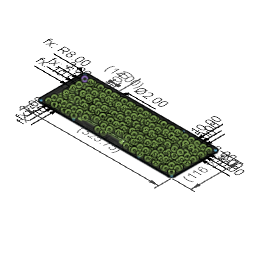
KeychronK6_Case (Autodesk Fusion 360 design; units mm, degrees)
Autodesk Fusion 360 part; units mm, degrees
(part 1 of 4)
sketch "switch-plate" plane through (0, 0, 0) normal (0, 0, 1) x (1, 0, 0) in component "switch-plate"
  spline S0 degree 3 poles (280.7, -89.8) (280.7, -89.9104) (280.6104, -90) (280.5, -90) knots 0 0 0 0 1 1 1 1
  line L0 (280.5, -90) -> (266.9, -90)
  spline S1 degree 3 poles (266.9, -90) (266.7896, -90) (266.7, -89.9104) (266.7, -89.8) knots 2 2 2 2 3 3 3 3
  line L1 (266.7, -89.8) -> (266.7, -76.2)
  spline S2 degree 3 poles (266.7, -76.2) (266.7, -76.0895) (266.7896, -76) (266.9, -76) knots 4 4 4 4 5 5 5 5
  line L2 (266.9, -76) -> (280.5, -76)
  spline S3 degree 3 poles (280.5, -76) (280.6104, -76) (280.7, -76.0895) (280.7, -76.2) knots 6 6 6 6 7 7 7 7
  line L3 (280.7, -76.2) -> (280.7, -89.8)
  spline S4 degree 3 poles (299.75, -13.6) (299.75, -13.7104) (299.6604, -13.8) (299.55, -13.8) knots 0 0 0 0 1 1 1 1
  line L4 (299.55, -13.8) -> (285.95, -13.8)
  spline S5 degree 3 poles (285.95, -13.8) (285.8396, -13.8) (285.75, -13.7104) (285.75, -13.6) knots 2 2 2 2 3 3 3 3
  line L5 (285.75, -13.6) -> (285.75, 0)
  spline S6 degree 3 poles (285.75, 0) (285.75, 0.1105) (285.8396, 0.2) (285.95, 0.2) knots 4 4 4 4 5 5 5 5
  line L6 (285.95, 0.2) -> (299.55, 0.2)
  spline S7 degree 3 poles (299.55, 0.2) (299.6604, 0.2) (299.75, 0.1105) (299.75, 0) knots 6 6 6 6 7 7 7 7
  line L7 (299.75, 0) -> (299.75, -13.6)
  spline S8 degree 3 poles (228.3101, -70.75) (228.3101, -70.8604) (228.2205, -70.95) (228.1101, -70.95) knots 0 0 0 0 1 1 1 1
  line L8 (228.1101, -70.95) -> (214.5101, -70.95)
  spline S9 degree 3 poles (214.5101, -70.95) (214.3997, -70.95) (214.3101, -70.8604) (214.3101, -70.75) knots 2 2 2 2 3 3 3 3
  line L9 (214.3101, -70.75) -> (214.3101, -57.15)
  spline S10 degree 3 poles (214.3101, -57.15) (214.3101, -57.0395) (214.3997, -56.95) (214.5101, -56.95) knots 4 4 4 4 5 5 5 5
  line L10 (214.5101, -56.95) -> (228.1101, -56.95)
  spline S11 degree 3 poles (228.1101, -56.95) (228.2205, -56.95) (228.3101, -57.0395) (228.3101, -57.15) knots 6 6 6 6 7 7 7 7
  line L11 (228.3101, -57.15) -> (228.3101, -70.75)
  spline S12 degree 3 poles (261.65, -89.8) (261.65, -89.9104) (261.5604, -90) (261.45, -90) knots 0 0 0 0 1 1 1 1
  line L12 (261.45, -90) -> (247.85, -90)
  spline S13 degree 3 poles (247.85, -90) (247.7396, -90) (247.65, -89.9104) (247.65, -89.8) knots 2 2 2 2 3 3 3 3
  line L13 (247.65, -89.8) -> (247.65, -76.2)
  spline S14 degree 3 poles (247.65, -76.2) (247.65, -76.0895) (247.7396, -76) (247.85, -76) knots 4 4 4 4 5 5 5 5
  line L14 (247.85, -76) -> (261.45, -76)
  spline S15 degree 3 poles (261.45, -76) (261.5604, -76) (261.65, -76.0895) (261.65, -76.2) knots 6 6 6 6 7 7 7 7
  line L15 (261.65, -76.2) -> (261.65, -89.8)
  spline S16 degree 3 poles (242.6, -89.8) (242.6, -89.9104) (242.5104, -90) (242.4, -90) knots 0 0 0 0 1 1 1 1
  line L16 (242.4, -90) -> (228.8, -90)
  spline S17 degree 3 poles (228.8, -90) (228.6896, -90) (228.6, -89.9104) (228.6, -89.8) knots 2 2 2 2 3 3 3 3
  line L17 (228.6, -89.8) -> (228.6, -76.2)
  spline S18 degree 3 poles (228.6, -76.2) (228.6, -76.0895) (228.6896, -76) (228.8, -76) knots 4 4 4 4 5 5 5 5
  line L18 (228.8, -76) -> (242.4, -76)
  spline S19 degree 3 poles (242.4, -76) (242.5104, -76) (242.6, -76.0895) (242.6, -76.2) knots 6 6 6 6 7 7 7 7
  line L19 (242.6, -76.2) -> (242.6, -89.8)
  spline S20 degree 3 poles (280.7, -70.75) (280.7, -70.8604) (280.6104, -70.95) (280.5, -70.95) knots 0 0 0 0 1 1 1 1
  line L20 (280.5, -70.95) -> (266.9, -70.95)
  spline S21 degree 3 poles (266.9, -70.95) (266.7896, -70.95) (266.7, -70.8604) (266.7, -70.75) knots 2 2 2 2 3 3 3 3
  line L21 (266.7, -70.75) -> (266.7, -57.15)
  spline S22 degree 3 poles (266.7, -57.15) (266.7, -57.0395) (266.7896, -56.95) (266.9, -56.95) knots 4 4 4 4 5 5 5 5
  line L22 (266.9, -56.95) -> (280.5, -56.95)
  spline S23 degree 3 poles (280.5, -56.95) (280.6104, -56.95) (280.7, -57.0395) (280.7, -57.15) knots 6 6 6 6 7 7 7 7
  line L23 (280.7, -57.15) -> (280.7, -70.75)
  line L24 (304.75, 13.2) -> (-5, 13.2)
  line L25 (-13, 5.2) -> (-13, -95)
  line L26 (-5, -103) -> (304.75, -103)
  line L27 (312.75, -95) -> (312.75, 5.2)
  spline S24 degree 3 poles (299.75, -32.65) (299.75, -32.7604) (299.6604, -32.85) (299.55, -32.85) knots 0 0 0 0 1 1 1 1
  line L28 (299.55, -32.85) -> (285.95, -32.85)
  spline S25 degree 3 poles (285.95, -32.85) (285.8396, -32.85) (285.75, -32.7604) (285.75, -32.65) knots 2 2 2 2 3 3 3 3
  line L29 (285.75, -32.65) -> (285.75, -19.05)
  spline S26 degree 3 poles (285.75, -19.05) (285.75, -18.9395) (285.8396, -18.85) (285.95, -18.85) knots 4 4 4 4 5 5 5 5
  line L30 (285.95, -18.85) -> (299.55, -18.85)
  spline S27 degree 3 poles (299.55, -18.85) (299.6604, -18.85) (299.75, -18.9395) (299.75, -19.05) knots 6 6 6 6 7 7 7 7
  line L31 (299.75, -19.05) -> (299.75, -32.65)
  spline S28 degree 3 poles (299.75, -70.75) (299.75, -70.8604) (299.6604, -70.95) (299.55, -70.95) knots 0 0 0 0 1 1 1 1
  line L32 (299.55, -70.95) -> (285.95, -70.95)
  spline S29 degree 3 poles (285.95, -70.95) (285.8396, -70.95) (285.75, -70.8604) (285.75, -70.75) knots 2 2 2 2 3 3 3 3
  line L33 (285.75, -70.75) -> (285.75, -57.15)
  spline S30 degree 3 poles (285.75, -57.15) (285.75, -57.0395) (285.8396, -56.95) (285.95, -56.95) knots 4 4 4 4 5 5 5 5
  line L34 (285.95, -56.95) -> (299.55, -56.95)
  spline S31 degree 3 poles (299.55, -56.95) (299.6604, -56.95) (299.75, -57.0395) (299.75, -57.15) knots 6 6 6 6 7 7 7 7
  line L35 (299.75, -57.15) -> (299.75, -70.75)
  spline S32 degree 3 poles (299.75, -89.8) (299.75, -89.9104) (299.6604, -90) (299.55, -90) knots 0 0 0 0 1 1 1 1
  line L36 (299.55, -90) -> (285.95, -90)
  spline S33 degree 3 poles (285.95, -90) (285.8396, -90) (285.75, -89.9104) (285.75, -89.8) knots 2 2 2 2 3 3 3 3
  line L37 (285.75, -89.8) -> (285.75, -76.2)
  spline S34 degree 3 poles (285.75, -76.2) (285.75, -76.0895) (285.8396, -76) (285.95, -76) knots 4 4 4 4 5 5 5 5
  line L38 (285.95, -76) -> (299.55, -76)
  spline S35 degree 3 poles (299.55, -76) (299.6604, -76) (299.75, -76.0895) (299.75, -76.2) knots 6 6 6 6 7 7 7 7
  line L39 (299.75, -76.2) -> (299.75, -89.8)
  spline S36 degree 3 poles (299.75, -51.7) (299.75, -51.8104) (299.6604, -51.9) (299.55, -51.9) knots 0 0 0 0 1 1 1 1
  line L40 (299.55, -51.9) -> (285.95, -51.9)
  spline S37 degree 3 poles (285.95, -51.9) (285.8396, -51.9) (285.75, -51.8104) (285.75, -51.7) knots 2 2 2 2 3 3 3 3
  line L41 (285.75, -51.7) -> (285.75, -38.1)
  spline S38 degree 3 poles (285.75, -38.1) (285.75, -37.9895) (285.8396, -37.9) (285.95, -37.9) knots 4 4 4 4 5 5 5 5
  line L42 (285.95, -37.9) -> (299.55, -37.9)
  spline S39 degree 3 poles (299.55, -37.9) (299.6604, -37.9) (299.75, -37.9895) (299.75, -38.1) knots 6 6 6 6 7 7 7 7
  line L43 (299.75, -38.1) -> (299.75, -51.7)
  spline S40 degree 3 poles (228.6, 0) (228.6, 0.1105) (228.6896, 0.2) (228.8, 0.2) knots 0 0 0 0 1 1 1 1
  line L44 (228.8, 0.2) -> (242.4, 0.2)
  spline S41 degree 3 poles (242.4, 0.2) (242.5104, 0.2) (242.6, 0.1105) (242.6, 0) knots 2 2 2 2 3 3 3 3
  line L45 (242.6, 0) -> (242.6, -13.6)
  spline S42 degree 3 poles (242.6, -13.6) (242.6, -13.7104) (242.5104, -13.8) (242.4, -13.8) knots 4 4 4 4 5 5 5 5
  line L46 (242.4, -13.8) -> (228.8, -13.8)
  spline S43 degree 3 poles (228.8, -13.8) (228.6896, -13.8) (228.6, -13.7104) (228.6, -13.6) knots 6 6 6 6 7 7 7 7
  line L47 (228.6, -13.6) -> (228.6, 0)
  spline S44 degree 3 poles (238.3302, -32.85) (238.2196, -32.85) (238.13, -32.7604) (238.13, -32.65) knots 0 0 0 0 1 1 1 1
  line L48 (238.13, -32.65) -> (238.13, -19.05)
  spline S45 degree 3 poles (238.13, -19.05) (238.13, -18.9395) (238.2196, -18.85) (238.3302, -18.85) knots 2 2 2 2 3 3 3 3
  line L49 (238.3302, -18.85) -> (251.93, -18.85)
  spline S46 degree 3 poles (251.93, -18.85) (252.0406, -18.85) (252.13, -18.9395) (252.13, -19.05) knots 4 4 4 4 5 5 5 5
  line L50 (252.13, -19.05) -> (252.13, -32.65)
  spline S47 degree 3 poles (252.13, -32.65) (252.13, -32.7604) (252.0406, -32.85) (251.93, -32.85) knots 6 6 6 6 7 7 7 7
  line L51 (251.93, -32.85) -> (238.3302, -32.85)
  line L52 (261.9401, -32.65) -> (261.9401, -19.05)
  spline S48 degree 3 poles (261.9401, -19.05) (261.9401, -18.9395) (262.0297, -18.85) (262.1401, -18.85) knots 1 1 1 1 2 2 2 2
  line L53 (262.1401, -18.85) -> (275.7401, -18.85)
  spline S49 degree 3 poles (275.7401, -18.85) (275.8505, -18.85) (275.9401, -18.9395) (275.9401, -19.05) knots 3 3 3 3 4 4 4 4
  line L54 (275.9401, -19.05) -> (275.9401, -32.65)
  spline S50 degree 3 poles (275.9401, -32.65) (275.9401, -32.7604) (275.8505, -32.85) (275.7401, -32.85) knots 5 5 5 5 6 6 6 6
  line L55 (275.7401, -32.85) -> (262.1401, -32.85)
  spline S51 degree 3 poles (262.1401, -32.85) (262.0297, -32.85) (261.9401, -32.7604) (261.9401, -32.65) knots 7 7 7 7 8 8 8 8
  spline S52 degree 3 poles (219.2802, -32.85) (219.1696, -32.85) (219.08, -32.7604) (219.08, -32.65) knots 0 0 0 0 1 1 1 1
  line L56 (219.08, -32.65) -> (219.08, -19.05)
  spline S53 degree 3 poles (219.08, -19.05) (219.08, -18.9395) (219.1696, -18.85) (219.2802, -18.85) knots 2 2 2 2 3 3 3 3
  line L57 (219.2802, -18.85) -> (232.88, -18.85)
  spline S54 degree 3 poles (232.88, -18.85) (232.9906, -18.85) (233.08, -18.9395) (233.08, -19.05) knots 4 4 4 4 5 5 5 5
  line L58 (233.08, -19.05) -> (233.08, -32.65)
  spline S55 degree 3 poles (233.08, -32.65) (233.08, -32.7604) (232.9906, -32.85) (232.88, -32.85) knots 6 6 6 6 7 7 7 7
  line L59 (232.88, -32.85) -> (219.2802, -32.85)
  spline S56 degree 3 poles (223.8301, -38.1) (223.8301, -37.9895) (223.9197, -37.9) (224.0301, -37.9) knots 0 0 0 0 1 1 1 1
  line L60 (224.0301, -37.9) -> (237.6301, -37.9)
  spline S57 degree 3 poles (237.6301, -37.9) (237.7405, -37.9) (237.8301, -37.9895) (237.8301, -38.1) knots 2 2 2 2 3 3 3 3
  line L61 (237.8301, -38.1) -> (237.8301, -51.7)
  spline S58 degree 3 poles (237.8301, -51.7) (237.8301, -51.8104) (237.7405, -51.9) (237.6301, -51.9) knots 4 4 4 4 5 5 5 5
  line L62 (237.6301, -51.9) -> (224.0301, -51.9)
  spline S59 degree 3 poles (224.0301, -51.9) (223.9197, -51.9) (223.8301, -51.8104) (223.8301, -51.7) knots 6 6 6 6 7 7 7 7
  line L63 (223.8301, -51.7) -> (223.8301, -38.1)
  line L64 (248.0298, -4.32) -> (248.8547, -4.32)
  line L65 (248.8547, -4.32) -> (248.8547, -1.32)
  line L66 (248.8547, -1.32) -> (255.5046, -1.32)
  line L67 (255.5046, -1.32) -> (255.5046, -3.82)
  line L68 (255.5046, -3.82) -> (257.18, -3.82)
  line L69 (257.18, -3.82) -> (257.18, 0)
  spline S60 degree 3 poles (257.18, 0) (257.18, 0.1105) (257.2696, 0.2) (257.3802, 0.2) knots 6 6 6 6 7 7 7 7
  line L70 (257.3802, 0.2) -> (270.98, 0.2)
  spline S61 degree 3 poles (270.98, 0.2) (271.0906, 0.2) (271.18, 0.1105) (271.18, 0) knots 8 8 8 8 9 9 9 9
  line L71 (271.18, 0) -> (271.18, -3.82)
  line L72 (271.18, -3.82) -> (272.8557, -3.82)
  line L73 (272.8557, -3.82) -> (272.8557, -1.32)
  line L74 (272.8557, -1.32) -> (279.5058, -1.32)
  line L75 (279.5058, -1.32) -> (279.5058, -4.32)
  line L76 (279.5058, -4.32) -> (280.3307, -4.32)
  line L77 (280.3307, -4.32) -> (280.3307, -7.33)
  line L78 (280.3307, -7.33) -> (279.5058, -7.33)
  line L79 (279.5058, -7.33) -> (279.5058, -13.53)
  line L80 (279.5058, -13.53) -> (277.6807, -13.53)
  line L81 (277.6807, -13.53) -> (277.6807, -14.78)
  line L82 (277.6807, -14.78) -> (274.6807, -14.78)
  line L83 (274.6807, -14.78) -> (274.6807, -13.53)
  line L84 (274.6807, -13.53) -> (272.8557, -13.53)
  line L85 (272.8557, -13.53) -> (272.8557, -11.03)
  line L86 (272.8557, -11.03) -> (271.18, -11.03)
  line L87 (271.18, -11.03) -> (271.18, -13.6)
  spline S62 degree 3 poles (271.18, -13.6) (271.18, -13.7104) (271.0906, -13.8) (270.98, -13.8) knots 26 26 26 26 27 27 27 27
  line L88 (270.98, -13.8) -> (257.3802, -13.8)
  spline S63 degree 3 poles (257.3802, -13.8) (257.2696, -13.8) (257.18, -13.7104) (257.18, -13.6) knots 28 28 28 28 29 29 29 29
  line L89 (257.18, -13.6) -> (257.18, -11.03)
  line L90 (257.18, -11.03) -> (255.5046, -11.03)
  line L91 (255.5046, -11.03) -> (255.5046, -13.53)
  line L92 (255.5046, -13.53) -> (253.6798, -13.53)
  line L93 (253.6798, -13.53) -> (253.6798, -14.78)
  line L94 (253.6798, -14.78) -> (250.6798, -14.78)
  line L95 (250.6798, -14.78) -> (250.6798, -13.53)
  line L96 (250.6798, -13.53) -> (248.8547, -13.53)
  line L97 (248.8547, -13.53) -> (248.8547, -7.33)
  line L98 (248.8547, -7.33) -> (248.0298, -7.33)
  line L99 (248.0298, -7.33) -> (248.0298, -4.32)
  spline S64 degree 3 poles (240.505, -57.15) (240.505, -57.0395) (240.5946, -56.95) (240.705, -56.95) knots 0 0 0 0 1 1 1 1
  line L100 (240.705, -56.95) -> (254.3051, -56.95)
  spline S65 degree 3 poles (254.3051, -56.95) (254.4155, -56.95) (254.5051, -57.0395) (254.5051, -57.15) knots 2 2 2 2 3 3 3 3
  line L101 (254.5051, -57.15) -> (254.5051, -70.75)
  spline S66 degree 3 poles (254.5051, -70.75) (254.5051, -70.8604) (254.4155, -70.95) (254.3051, -70.95) knots 4 4 4 4 5 5 5 5
  line L102 (254.3051, -70.95) -> (240.705, -70.95)
  spline S67 degree 3 poles (240.705, -70.95) (240.5946, -70.95) (240.505, -70.8604) (240.505, -70.75) knots 6 6 6 6 7 7 7 7
  line L103 (240.505, -70.75) -> (240.505, -57.15)
  line L104 (270.4557, -51.63) -> (270.4557, -49.13)
  line L105 (270.4557, -49.13) -> (268.78, -49.13)
  line L106 (268.78, -49.13) -> (268.78, -51.7)
  spline S68 degree 3 poles (268.78, -51.7) (268.78, -51.8104) (268.6906, -51.9) (268.5802, -51.9) knots 3 3 3 3 4 4 4 4
  line L107 (268.5802, -51.9) -> (254.9801, -51.9)
  spline S69 degree 3 poles (254.9801, -51.9) (254.8695, -51.9) (254.7801, -51.8104) (254.7801, -51.7) knots 5 5 5 5 6 6 6 6
  line L108 (254.7801, -51.7) -> (254.7801, -49.13)
  line L109 (254.7801, -49.13) -> (253.1046, -49.13)
  line L110 (253.1046, -49.13) -> (253.1046, -51.63)
  line L111 (253.1046, -51.63) -> (251.2798, -51.63)
  line L112 (251.2798, -51.63) -> (251.2798, -52.88)
  line L113 (251.2798, -52.88) -> (248.2798, -52.88)
  line L114 (248.2798, -52.88) -> (248.2798, -51.63)
  line L115 (248.2798, -51.63) -> (246.4547, -51.63)
  line L116 (246.4547, -51.63) -> (246.4547, -45.43)
  line L117 (246.4547, -45.43) -> (245.6298, -45.43)
  line L118 (245.6298, -45.43) -> (245.6298, -42.42)
  line L119 (245.6298, -42.42) -> (246.4547, -42.42)
  line L120 (246.4547, -42.42) -> (246.4547, -39.42)
  line L121 (246.4547, -39.42) -> (253.1046, -39.42)
  line L122 (253.1046, -39.42) -> (253.1046, -41.92)
  line L123 (253.1046, -41.92) -> (254.7801, -41.92)
  line L124 (254.7801, -41.92) -> (254.7801, -38.1)
  spline S70 degree 3 poles (254.7801, -38.1) (254.7801, -37.9895) (254.8695, -37.9) (254.9801, -37.9) knots 23 23 23 23 24 24 24 24
  line L125 (254.9801, -37.9) -> (268.5802, -37.9)
  spline S71 degree 3 poles (268.5802, -37.9) (268.6906, -37.9) (268.78, -37.9895) (268.78, -38.1) knots 25 25 25 25 26 26 26 26
  line L126 (268.78, -38.1) -> (268.78, -41.92)
  line L127 (268.78, -41.92) -> (270.4557, -41.92)
  line L128 (270.4557, -41.92) -> (270.4557, -39.42)
  line L129 (270.4557, -39.42) -> (277.1057, -39.42)
  line L130 (277.1057, -39.42) -> (277.1057, -42.42)
  line L131 (277.1057, -42.42) -> (277.9307, -42.42)
  line L132 (277.9307, -42.42) -> (277.9307, -45.43)
  line L133 (277.9307, -45.43) -> (277.1057, -45.43)
  line L134 (277.1057, -45.43) -> (277.1057, -51.63)
  line L135 (277.1057, -51.63) -> (275.2807, -51.63)
  line L136 (275.2807, -51.63) -> (275.2807, -52.88)
  line L137 (275.2807, -52.88) -> (272.2807, -52.88)
  line L138 (272.2807, -52.88) -> (272.2807, -51.63)
  line L139 (272.2807, -51.63) -> (270.4557, -51.63)
  spline S72 degree 3 poles (147.8301, -51.9) (147.7197, -51.9) (147.6301, -51.8104) (147.6301, -51.7) knots 0 0 0 0 1 1 1 1
  line L140 (147.6301, -51.7) -> (147.6301, -38.1)
  spline S73 degree 3 poles (147.6301, -38.1) (147.6301, -37.9895) (147.7197, -37.9) (147.8301, -37.9) knots 2 2 2 2 3 3 3 3
  line L141 (147.8301, -37.9) -> (161.4301, -37.9)
  spline S74 degree 3 poles (161.4301, -37.9) (161.5405, -37.9) (161.6301, -37.9895) (161.6301, -38.1) knots 4 4 4 4 5 5 5 5
  line L142 (161.6301, -38.1) -> (161.6301, -51.7)
  spline S75 degree 3 poles (161.6301, -51.7) (161.6301, -51.8104) (161.5405, -51.9) (161.4301, -51.9) knots 6 6 6 6 7 7 7 7
  line L143 (161.4301, -51.9) -> (147.8301, -51.9)
  line L144 (142.88, -32.65) -> (142.88, -19.05)
  spline S76 degree 3 poles (142.88, -19.05) (142.88, -18.9395) (142.9696, -18.85) (143.0802, -18.85) knots 1 1 1 1 2 2 2 2
  line L145 (143.0802, -18.85) -> (156.68, -18.85)
  spline S77 degree 3 poles (156.68, -18.85) (156.7906, -18.85) (156.88, -18.9395) (156.88, -19.05) knots 3 3 3 3 4 4 4 4
  line L146 (156.88, -19.05) -> (156.88, -32.65)
  spline S78 degree 3 poles (156.88, -32.65) (156.88, -32.7604) (156.7906, -32.85) (156.68, -32.85) knots 5 5 5 5 6 6 6 6
  line L147 (156.68, -32.85) -> (143.0802, -32.85)
  spline S79 degree 3 poles (143.0802, -32.85) (142.9696, -32.85) (142.88, -32.7604) (142.88, -32.65) knots 7 7 7 7 8 8 8 8
  spline S80 degree 3 poles (157.1601, -57.15) (157.1601, -57.0395) (157.2497, -56.95) (157.3601, -56.95) knots 0 0 0 0 1 1 1 1
  line L148 (157.3601, -56.95) -> (170.9601, -56.95)
  spline S81 degree 3 poles (170.9601, -56.95) (171.0705, -56.95) (171.1601, -57.0395) (171.1601, -57.15) knots 2 2 2 2 3 3 3 3
  line L149 (171.1601, -57.15) -> (171.1601, -70.75)
  spline S82 degree 3 poles (171.1601, -70.75) (171.1601, -70.8604) (171.0705, -70.95) (170.9601, -70.95) knots 4 4 4 4 5 5 5 5
  line L150 (170.9601, -70.95) -> (157.3601, -70.95)
  spline S83 degree 3 poles (157.3601, -70.95) (157.2497, -70.95) (157.1601, -70.8604) (157.1601, -70.75) knots 6 6 6 6 7 7 7 7
  line L151 (157.1601, -70.75) -> (157.1601, -57.15)
  spline S84 degree 3 poles (166.8801, -51.9) (166.7697, -51.9) (166.6801, -51.8104) (166.6801, -51.7) knots 0 0 0 0 1 1 1 1
  line L152 (166.6801, -51.7) -> (166.6801, -38.1)
  spline S85 degree 3 poles (166.6801, -38.1) (166.6801, -37.9895) (166.7697, -37.9) (166.8801, -37.9) knots 2 2 2 2 3 3 3 3
  line L153 (166.8801, -37.9) -> (180.4801, -37.9)
  spline S86 degree 3 poles (180.4801, -37.9) (180.5905, -37.9) (180.6801, -37.9895) (180.6801, -38.1) knots 4 4 4 4 5 5 5 5
  line L154 (180.6801, -38.1) -> (180.6801, -51.7)
  spline S87 degree 3 poles (180.6801, -51.7) (180.6801, -51.8104) (180.5905, -51.9) (180.4801, -51.9) knots 6 6 6 6 7 7 7 7
  line L155 (180.4801, -51.9) -> (166.8801, -51.9)
  line L156 (104.78, -32.65) -> (104.78, -19.05)
  spline S88 degree 3 poles (104.78, -19.05) (104.78, -18.9395) (104.8696, -18.85) (104.9802, -18.85) knots 1 1 1 1 2 2 2 2
  line L157 (104.9802, -18.85) -> (118.58, -18.85)
  spline S89 degree 3 poles (118.58, -18.85) (118.6906, -18.85) (118.78, -18.9395) (118.78, -19.05) knots 3 3 3 3 4 4 4 4
  line L158 (118.78, -19.05) -> (118.78, -32.65)
  spline S90 degree 3 poles (118.78, -32.65) (118.78, -32.7604) (118.6906, -32.85) (118.58, -32.85) knots 5 5 5 5 6 6 6 6
  line L159 (118.58, -32.85) -> (104.9802, -32.85)
  spline S91 degree 3 poles (104.9802, -32.85) (104.8696, -32.85) (104.78, -32.7604) (104.78, -32.65) knots 7 7 7 7 8 8 8 8
  line L160 (161.93, -32.65) -> (161.93, -19.05)
  spline S92 degree 3 poles (161.93, -19.05) (161.93, -18.9395) (162.0196, -18.85) (162.1302, -18.85) knots 1 1 1 1 2 2 2 2
  line L161 (162.1302, -18.85) -> (175.73, -18.85)
  spline S93 degree 3 poles (175.73, -18.85) (175.8406, -18.85) (175.93, -18.9395) (175.93, -19.05) knots 3 3 3 3 4 4 4 4
  line L162 (175.93, -19.05) -> (175.93, -32.65)
  spline S94 degree 3 poles (175.93, -32.65) (175.93, -32.7604) (175.8406, -32.85) (175.73, -32.85) knots 5 5 5 5 6 6 6 6
  line L163 (175.73, -32.85) -> (162.1302, -32.85)
  spline S95 degree 3 poles (162.1302, -32.85) (162.0196, -32.85) (161.93, -32.7604) (161.93, -32.65) knots 7 7 7 7 8 8 8 8
  line L164 (85.73, -32.65) -> (85.73, -19.05)
  spline S96 degree 3 poles (85.73, -19.05) (85.73, -18.9395) (85.8196, -18.85) (85.9302, -18.85) knots 1 1 1 1 2 2 2 2
  line L165 (85.9302, -18.85) -> (99.53, -18.85)
  spline S97 degree 3 poles (99.53, -18.85) (99.6406, -18.85) (99.73, -18.9395) (99.73, -19.05) knots 3 3 3 3 4 4 4 4
  line L166 (99.73, -19.05) -> (99.73, -32.65)
  spline S98 degree 3 poles (99.73, -32.65) (99.73, -32.7604) (99.6406, -32.85) (99.53, -32.85) knots 5 5 5 5 6 6 6 6
  line L167 (99.53, -32.85) -> (85.9302, -32.85)
  spline S99 degree 3 poles (85.9302, -32.85) (85.8196, -32.85) (85.73, -32.7604) (85.73, -32.65) knots 7 7 7 7 8 8 8 8
  spline S100 degree 3 poles (200.2302, -32.85) (200.1196, -32.85) (200.03, -32.7604) (200.03, -32.65) knots 0 0 0 0 1 1 1 1
  line L168 (200.03, -32.65) -> (200.03, -19.05)
  spline S101 degree 3 poles (200.03, -19.05) (200.03, -18.9395) (200.1196, -18.85) (200.2302, -18.85) knots 2 2 2 2 3 3 3 3
  line L169 (200.2302, -18.85) -> (213.83, -18.85)
  spline S102 degree 3 poles (213.83, -18.85) (213.9406, -18.85) (214.03, -18.9395) (214.03, -19.05) knots 4 4 4 4 5 5 5 5
  line L170 (214.03, -19.05) -> (214.03, -32.65)
  spline S103 degree 3 poles (214.03, -32.65) (214.03, -32.7604) (213.9406, -32.85) (213.83, -32.85) knots 6 6 6 6 7 7 7 7
  line L171 (213.83, -32.85) -> (200.2302, -32.85)
  spline S104 degree 3 poles (171.45, 0) (171.45, 0.1105) (171.5396, 0.2) (171.65, 0.2) knots 0 0 0 0 1 1 1 1
  line L172 (171.65, 0.2) -> (185.25, 0.2)
  spline S105 degree 3 poles (185.25, 0.2) (185.3604, 0.2) (185.45, 0.1105) (185.45, 0) knots 2 2 2 2 3 3 3 3
  line L173 (185.45, 0) -> (185.45, -13.6)
  spline S106 degree 3 poles (185.45, -13.6) (185.45, -13.7104) (185.3604, -13.8) (185.25, -13.8) knots 4 4 4 4 5 5 5 5
  line L174 (185.25, -13.8) -> (171.65, -13.8)
  spline S107 degree 3 poles (171.65, -13.8) (171.5396, -13.8) (171.45, -13.7104) (171.45, -13.6) knots 6 6 6 6 7 7 7 7
  line L175 (171.45, -13.6) -> (171.45, 0)
  spline S108 degree 3 poles (138.1101, -57.15) (138.1101, -57.0395) (138.1997, -56.95) (138.3101, -56.95) knots 0 0 0 0 1 1 1 1
  line L176 (138.3101, -56.95) -> (151.9101, -56.95)
  spline S109 degree 3 poles (151.9101, -56.95) (152.0205, -56.95) (152.1101, -57.0395) (152.1101, -57.15) knots 2 2 2 2 3 3 3 3
  line L177 (152.1101, -57.15) -> (152.1101, -70.75)
  spline S110 degree 3 poles (152.1101, -70.75) (152.1101, -70.8604) (152.0205, -70.95) (151.9101, -70.95) knots 4 4 4 4 5 5 5 5
  line L178 (151.9101, -70.95) -> (138.3101, -70.95)
  spline S111 degree 3 poles (138.3101, -70.95) (138.1997, -70.95) (138.1101, -70.8604) (138.1101, -70.75) knots 6 6 6 6 7 7 7 7
  line L179 (138.1101, -70.75) -> (138.1101, -57.15)
  spline S112 degree 3 poles (52.3801, -38.1) (52.3801, -37.9895) (52.4697, -37.9) (52.5801, -37.9) knots 0 0 0 0 1 1 1 1
  line L180 (52.5801, -37.9) -> (66.1801, -37.9)
  spline S113 degree 3 poles (66.1801, -37.9) (66.2905, -37.9) (66.3801, -37.9895) (66.3801, -38.1) knots 2 2 2 2 3 3 3 3
  line L181 (66.3801, -38.1) -> (66.3801, -51.7)
  spline S114 degree 3 poles (66.3801, -51.7) (66.3801, -51.8104) (66.2905, -51.9) (66.1801, -51.9) knots 4 4 4 4 5 5 5 5
  line L182 (66.1801, -51.9) -> (52.5801, -51.9)
  spline S115 degree 3 poles (52.5801, -51.9) (52.4697, -51.9) (52.3801, -51.8104) (52.3801, -51.7) knots 6 6 6 6 7 7 7 7
  line L183 (52.3801, -51.7) -> (52.3801, -38.1)
  line L184 (66.68, -32.65) -> (66.68, -19.05)
  spline S116 degree 3 poles (66.68, -19.05) (66.68, -18.9395) (66.7696, -18.85) (66.8802, -18.85) knots 1 1 1 1 2 2 2 2
  line L185 (66.8802, -18.85) -> (80.48, -18.85)
  spline S117 degree 3 poles (80.48, -18.85) (80.5906, -18.85) (80.68, -18.9395) (80.68, -19.05) knots 3 3 3 3 4 4 4 4
  line L186 (80.68, -19.05) -> (80.68, -32.65)
  spline S118 degree 3 poles (80.68, -32.65) (80.68, -32.7604) (80.5906, -32.85) (80.48, -32.85) knots 5 5 5 5 6 6 6 6
  line L187 (80.48, -32.85) -> (66.8802, -32.85)
  spline S119 degree 3 poles (66.8802, -32.85) (66.7696, -32.85) (66.68, -32.7604) (66.68, -32.65) knots 7 7 7 7 8 8 8 8
  spline S120 degree 3 poles (114.3, 0) (114.3, 0.1105) (114.3896, 0.2) (114.5, 0.2) knots 0 0 0 0 1 1 1 1
  line L188 (114.5, 0.2) -> (128.1, 0.2)
  spline S121 degree 3 poles (128.1, 0.2) (128.2104, 0.2) (128.3, 0.1105) (128.3, 0) knots 2 2 2 2 3 3 3 3
  line L189 (128.3, 0) -> (128.3, -13.6)
  spline S122 degree 3 poles (128.3, -13.6) (128.3, -13.7104) (128.2104, -13.8) (128.1, -13.8) knots 4 4 4 4 5 5 5 5
  line L190 (128.1, -13.8) -> (114.5, -13.8)
  spline S123 degree 3 poles (114.5, -13.8) (114.3896, -13.8) (114.3, -13.7104) (114.3, -13.6) knots 6 6 6 6 7 7 7 7
  line L191 (114.3, -13.6) -> (114.3, 0)
  spline S124 degree 3 poles (152.4, 0) (152.4, 0.1105) (152.4896, 0.2) (152.6, 0.2) knots 0 0 0 0 1 1 1 1
  line L192 (152.6, 0.2) -> (166.2, 0.2)
  spline S125 degree 3 poles (166.2, 0.2) (166.3104, 0.2) (166.4, 0.1105) (166.4, 0) knots 2 2 2 2 3 3 3 3
  line L193 (166.4, 0) -> (166.4, -13.6)
  spline S126 degree 3 poles (166.4, -13.6) (166.4, -13.7104) (166.3104, -13.8) (166.2, -13.8) knots 4 4 4 4 5 5 5 5
  line L194 (166.2, -13.8) -> (152.6, -13.8)
  spline S127 degree 3 poles (152.6, -13.8) (152.4896, -13.8) (152.4, -13.7104) (152.4, -13.6) knots 6 6 6 6 7 7 7 7
  line L195 (152.4, -13.6) -> (152.4, 0)
  spline S128 degree 3 poles (133.35, 0) (133.35, 0.1105) (133.4396, 0.2) (133.55, 0.2) knots 0 0 0 0 1 1 1 1
  line L196 (133.55, 0.2) -> (147.15, 0.2)
  spline S129 degree 3 poles (147.15, 0.2) (147.2604, 0.2) (147.35, 0.1105) (147.35, 0) knots 2 2 2 2 3 3 3 3
  line L197 (147.35, 0) -> (147.35, -13.6)
  spline S130 degree 3 poles (147.35, -13.6) (147.35, -13.7104) (147.2604, -13.8) (147.15, -13.8) knots 4 4 4 4 5 5 5 5
  line L198 (147.15, -13.8) -> (133.55, -13.8)
  spline S131 degree 3 poles (133.55, -13.8) (133.4396, -13.8) (133.35, -13.7104) (133.35, -13.6) knots 6 6 6 6 7 7 7 7
  line L199 (133.35, -13.6) -> (133.35, 0)
  spline S132 degree 3 poles (204.7801, -38.1) (204.7801, -37.9895) (204.8697, -37.9) (204.9801, -37.9) knots 0 0 0 0 1 1 1 1
  line L200 (204.9801, -37.9) -> (218.5801, -37.9)
  spline S133 degree 3 poles (218.5801, -37.9) (218.6905, -37.9) (218.7801, -37.9895) (218.7801, -38.1) knots 2 2 2 2 3 3 3 3
  line L201 (218.7801, -38.1) -> (218.7801, -51.7)
  spline S134 degree 3 poles (218.7801, -51.7) (218.7801, -51.8104) (218.6905, -51.9) (218.5801, -51.9) knots 4 4 4 4 5 5 5 5
  line L202 (218.5801, -51.9) -> (204.9801, -51.9)
  spline S135 degree 3 poles (204.9801, -51.9) (204.8697, -51.9) (204.7801, -51.8104) (204.7801, -51.7) knots 6 6 6 6 7 7 7 7
  line L203 (204.7801, -51.7) -> (204.7801, -38.1)
  spline S136 degree 3 poles (185.7301, -38.1) (185.7301, -37.9895) (185.8197, -37.9) (185.9301, -37.9) knots 0 0 0 0 1 1 1 1
  line L204 (185.9301, -37.9) -> (199.5301, -37.9)
  spline S137 degree 3 poles (199.5301, -37.9) (199.6405, -37.9) (199.7301, -37.9895) (199.7301, -38.1) knots 2 2 2 2 3 3 3 3
  line L205 (199.7301, -38.1) -> (199.7301, -51.7)
  spline S138 degree 3 poles (199.7301, -51.7) (199.7301, -51.8104) (199.6405, -51.9) (199.5301, -51.9) knots 4 4 4 4 5 5 5 5
  line L206 (199.5301, -51.9) -> (185.9301, -51.9)
  spline S139 degree 3 poles (185.9301, -51.9) (185.8197, -51.9) (185.7301, -51.8104) (185.7301, -51.7) knots 6 6 6 6 7 7 7 7
  line L207 (185.7301, -51.7) -> (185.7301, -38.1)
  spline S140 degree 3 poles (128.7801, -51.9) (128.6697, -51.9) (128.5801, -51.8104) (128.5801, -51.7) knots 0 0 0 0 1 1 1 1
  line L208 (128.5801, -51.7) -> (128.5801, -38.1)
  spline S141 degree 3 poles (128.5801, -38.1) (128.5801, -37.9895) (128.6697, -37.9) (128.7801, -37.9) knots 2 2 2 2 3 3 3 3
  line L209 (128.7801, -37.9) -> (142.3801, -37.9)
  spline S142 degree 3 poles (142.3801, -37.9) (142.4905, -37.9) (142.5801, -37.9895) (142.5801, -38.1) knots 4 4 4 4 5 5 5 5
  line L210 (142.5801, -38.1) -> (142.5801, -51.7)
  spline S143 degree 3 poles (142.5801, -51.7) (142.5801, -51.8104) (142.4905, -51.9) (142.3801, -51.9) knots 6 6 6 6 7 7 7 7
  line L211 (142.3801, -51.9) -> (128.7801, -51.9)
  spline S144 degree 3 poles (190.5, 0) (190.5, 0.1105) (190.5896, 0.2) (190.7, 0.2) knots 0 0 0 0 1 1 1 1
  line L212 (190.7, 0.2) -> (204.3, 0.2)
  spline S145 degree 3 poles (204.3, 0.2) (204.4104, 0.2) (204.5, 0.1105) (204.5, 0) knots 2 2 2 2 3 3 3 3
  line L213 (204.5, 0) -> (204.5, -13.6)
  spline S146 degree 3 poles (204.5, -13.6) (204.5, -13.7104) (204.4104, -13.8) (204.3, -13.8) knots 4 4 4 4 5 5 5 5
  line L214 (204.3, -13.8) -> (190.7, -13.8)
  spline S147 degree 3 poles (190.7, -13.8) (190.5896, -13.8) (190.5, -13.7104) (190.5, -13.6) knots 6 6 6 6 7 7 7 7
  line L215 (190.5, -13.6) -> (190.5, 0)
  spline S148 degree 3 poles (80.9601, -57.15) (80.9601, -57.0395) (81.0497, -56.95) (81.1601, -56.95) knots 0 0 0 0 1 1 1 1
  line L216 (81.1601, -56.95) -> (94.7601, -56.95)
  spline S149 degree 3 poles (94.7601, -56.95) (94.8705, -56.95) (94.9601, -57.0395) (94.9601, -57.15) knots 2 2 2 2 3 3 3 3
  line L217 (94.9601, -57.15) -> (94.9601, -70.75)
  spline S150 degree 3 poles (94.9601, -70.75) (94.9601, -70.8604) (94.8705, -70.95) (94.7601, -70.95) knots 4 4 4 4 5 5 5 5
  line L218 (94.7601, -70.95) -> (81.1601, -70.95)
  spline S151 degree 3 poles (81.1601, -70.95) (81.0497, -70.95) (80.9601, -70.8604) (80.9601, -70.75) knots 6 6 6 6 7 7 7 7
  line L219 (80.9601, -70.75) -> (80.9601, -57.15)
  spline S152 degree 3 poles (90.6801, -51.9) (90.5697, -51.9) (90.4801, -51.8104) (90.4801, -51.7) knots 0 0 0 0 1 1 1 1
  line L220 (90.4801, -51.7) -> (90.4801, -38.1)
  spline S153 degree 3 poles (90.4801, -38.1) (90.4801, -37.9895) (90.5697, -37.9) (90.6801, -37.9) knots 2 2 2 2 3 3 3 3
  line L221 (90.6801, -37.9) -> (104.2801, -37.9)
  spline S154 degree 3 poles (104.2801, -37.9) (104.3905, -37.9) (104.4801, -37.9895) (104.4801, -38.1) knots 4 4 4 4 5 5 5 5
  line L222 (104.4801, -38.1) -> (104.4801, -51.7)
  spline S155 degree 3 poles (104.4801, -51.7) (104.4801, -51.8104) (104.3905, -51.9) (104.2801, -51.9) knots 6 6 6 6 7 7 7 7
  line L223 (104.2801, -51.9) -> (90.6801, -51.9)
  line L224 (123.83, -32.65) -> (123.83, -19.05)
  spline S156 degree 3 poles (123.83, -19.05) (123.83, -18.9395) (123.9196, -18.85) (124.0302, -18.85) knots 1 1 1 1 2 2 2 2
  line L225 (124.0302, -18.85) -> (137.63, -18.85)
  spline S157 degree 3 poles (137.63, -18.85) (137.7406, -18.85) (137.83, -18.9395) (137.83, -19.05) knots 3 3 3 3 4 4 4 4
  line L226 (137.83, -19.05) -> (137.83, -32.65)
  spline S158 degree 3 poles (137.83, -32.65) (137.83, -32.7604) (137.7406, -32.85) (137.63, -32.85) knots 5 5 5 5 6 6 6 6
  line L227 (137.63, -32.85) -> (124.0302, -32.85)
  spline S159 degree 3 poles (124.0302, -32.85) (123.9196, -32.85) (123.83, -32.7604) (123.83, -32.65) knots 7 7 7 7 8 8 8 8
  spline S160 degree 3 poles (47.8302, -32.85) (47.7196, -32.85) (47.63, -32.7604) (47.63, -32.65) knots 0 0 0 0 1 1 1 1
  line L228 (47.63, -32.65) -> (47.63, -19.05)
  spline S161 degree 3 poles (47.63, -19.05) (47.63, -18.9395) (47.7196, -18.85) (47.8302, -18.85) knots 2 2 2 2 3 3 3 3
  line L229 (47.8302, -18.85) -> (61.43, -18.85)
  spline S162 degree 3 poles (61.43, -18.85) (61.5406, -18.85) (61.63, -18.9395) (61.63, -19.05) knots 4 4 4 4 5 5 5 5
  line L230 (61.63, -19.05) -> (61.63, -32.65)
  spline S163 degree 3 poles (61.63, -32.65) (61.63, -32.7604) (61.5406, -32.85) (61.43, -32.85) knots 6 6 6 6 7 7 7 7
  line L231 (61.43, -32.85) -> (47.8302, -32.85)
  spline S164 degree 3 poles (109.7301, -51.9) (109.6197, -51.9) (109.5301, -51.8104) (109.5301, -51.7) knots 0 0 0 0 1 1 1 1
  line L232 (109.5301, -51.7) -> (109.5301, -38.1)
  spline S165 degree 3 poles (109.5301, -38.1) (109.5301, -37.9895) (109.6197, -37.9) (109.7301, -37.9) knots 2 2 2 2 3 3 3 3
  line L233 (109.7301, -37.9) -> (123.3301, -37.9)
  spline S166 degree 3 poles (123.3301, -37.9) (123.4405, -37.9) (123.5301, -37.9895) (123.5301, -38.1) knots 4 4 4 4 5 5 5 5
  line L234 (123.5301, -38.1) -> (123.5301, -51.7)
  spline S167 degree 3 poles (123.5301, -51.7) (123.5301, -51.8104) (123.4405, -51.9) (123.3301, -51.9) knots 6 6 6 6 7 7 7 7
  line L235 (123.3301, -51.9) -> (109.7301, -51.9)
  spline S168 degree 3 poles (61.9101, -57.15) (61.9101, -57.0395) (61.9997, -56.95) (62.1101, -56.95) knots 0 0 0 0 1 1 1 1
  line L236 (62.1101, -56.95) -> (75.7101, -56.95)
  spline S169 degree 3 poles (75.7101, -56.95) (75.8205, -56.95) (75.9101, -57.0395) (75.9101, -57.15) knots 2 2 2 2 3 3 3 3
  line L237 (75.9101, -57.15) -> (75.9101, -70.75)
  spline S170 degree 3 poles (75.9101, -70.75) (75.9101, -70.8604) (75.8205, -70.95) (75.7101, -70.95) knots 4 4 4 4 5 5 5 5
  line L238 (75.7101, -70.95) -> (62.1101, -70.95)
  spline S171 degree 3 poles (62.1101, -70.95) (61.9997, -70.95) (61.9101, -70.8604) (61.9101, -70.75) knots 6 6 6 6 7 7 7 7
  line L239 (61.9101, -70.75) -> (61.9101, -57.15)
  spline S172 degree 3 poles (71.6301, -51.9) (71.5197, -51.9) (71.4301, -51.8104) (71.4301, -51.7) knots 0 0 0 0 1 1 1 1
  line L240 (71.4301, -51.7) -> (71.4301, -38.1)
  spline S173 degree 3 poles (71.4301, -38.1) (71.4301, -37.9895) (71.5197, -37.9) (71.6301, -37.9) knots 2 2 2 2 3 3 3 3
  line L241 (71.6301, -37.9) -> (85.2301, -37.9)
  spline S174 degree 3 poles (85.2301, -37.9) (85.3405, -37.9) (85.4301, -37.9895) (85.4301, -38.1) knots 4 4 4 4 5 5 5 5
  line L242 (85.4301, -38.1) -> (85.4301, -51.7)
  spline S175 degree 3 poles (85.4301, -51.7) (85.4301, -51.8104) (85.3405, -51.9) (85.2301, -51.9) knots 6 6 6 6 7 7 7 7
  line L243 (85.2301, -51.9) -> (71.6301, -51.9)
  spline S176 degree 3 poles (209.55, 0) (209.55, 0.1105) (209.6396, 0.2) (209.75, 0.2) knots 0 0 0 0 1 1 1 1
  line L244 (209.75, 0.2) -> (223.35, 0.2)
  spline S177 degree 3 poles (223.35, 0.2) (223.4604, 0.2) (223.55, 0.1105) (223.55, 0) knots 2 2 2 2 3 3 3 3
  line L245 (223.55, 0) -> (223.55, -13.6)
  spline S178 degree 3 poles (223.55, -13.6) (223.55, -13.7104) (223.4604, -13.8) (223.35, -13.8) knots 4 4 4 4 5 5 5 5
  line L246 (223.35, -13.8) -> (209.75, -13.8)
  spline S179 degree 3 poles (209.75, -13.8) (209.6396, -13.8) (209.55, -13.7104) (209.55, -13.6) knots 6 6 6 6 7 7 7 7
  line L247 (209.55, -13.6) -> (209.55, 0)
  spline S180 degree 3 poles (181.1802, -32.85) (181.0696, -32.85) (180.98, -32.7604) (180.98, -32.65) knots 0 0 0 0 1 1 1 1
  line L248 (180.98, -32.65) -> (180.98, -19.05)
  spline S181 degree 3 poles (180.98, -19.05) (180.98, -18.9395) (181.0696, -18.85) (181.1802, -18.85) knots 2 2 2 2 3 3 3 3
  line L249 (181.1802, -18.85) -> (194.78, -18.85)
  spline S182 degree 3 poles (194.78, -18.85) (194.8906, -18.85) (194.98, -18.9395) (194.98, -19.05) knots 4 4 4 4 5 5 5 5
  line L250 (194.98, -19.05) -> (194.98, -32.65)
  spline S183 degree 3 poles (194.98, -32.65) (194.98, -32.7604) (194.8906, -32.85) (194.78, -32.85) knots 6 6 6 6 7 7 7 7
  line L251 (194.78, -32.85) -> (181.1802, -32.85)
  spline S184 degree 3 poles (100.0101, -57.15) (100.0101, -57.0395) (100.0997, -56.95) (100.2101, -56.95) knots 0 0 0 0 1 1 1 1
  line L252 (100.2101, -56.95) -> (113.8101, -56.95)
  spline S185 degree 3 poles (113.8101, -56.95) (113.9205, -56.95) (114.0101, -57.0395) (114.0101, -57.15) knots 2 2 2 2 3 3 3 3
  line L253 (114.0101, -57.15) -> (114.0101, -70.75)
  spline S186 degree 3 poles (114.0101, -70.75) (114.0101, -70.8604) (113.9205, -70.95) (113.8101, -70.95) knots 4 4 4 4 5 5 5 5
  line L254 (113.8101, -70.95) -> (100.2101, -70.95)
  spline S187 degree 3 poles (100.2101, -70.95) (100.0997, -70.95) (100.0101, -70.8604) (100.0101, -70.75) knots 6 6 6 6 7 7 7 7
  line L255 (100.0101, -70.75) -> (100.0101, -57.15)
  spline S188 degree 3 poles (119.0601, -57.15) (119.0601, -57.0395) (119.1497, -56.95) (119.2601, -56.95) knots 0 0 0 0 1 1 1 1
  line L256 (119.2601, -56.95) -> (132.8601, -56.95)
  spline S189 degree 3 poles (132.8601, -56.95) (132.9705, -56.95) (133.0601, -57.0395) (133.0601, -57.15) knots 2 2 2 2 3 3 3 3
  line L257 (133.0601, -57.15) -> (133.0601, -70.75)
  spline S190 degree 3 poles (133.0601, -70.75) (133.0601, -70.8604) (132.9705, -70.95) (132.8601, -70.95) knots 4 4 4 4 5 5 5 5
  line L258 (132.8601, -70.95) -> (119.2601, -70.95)
  spline S191 degree 3 poles (119.2601, -70.95) (119.1497, -70.95) (119.0601, -70.8604) (119.0601, -70.75) knots 6 6 6 6 7 7 7 7
  line L259 (119.0601, -70.75) -> (119.0601, -57.15)
  line L260 (42.8601, -70.75) -> (42.8601, -57.15)
  spline S192 degree 3 poles (42.8601, -57.15) (42.8601, -57.0395) (42.9497, -56.95) (43.0601, -56.95) knots 1 1 1 1 2 2 2 2
  line L261 (43.0601, -56.95) -> (56.6601, -56.95)
  spline S193 degree 3 poles (56.6601, -56.95) (56.7705, -56.95) (56.8601, -57.0395) (56.8601, -57.15) knots 3 3 3 3 4 4 4 4
  line L262 (56.8601, -57.15) -> (56.8601, -70.75)
  spline S194 degree 3 poles (56.8601, -70.75) (56.8601, -70.8604) (56.7705, -70.95) (56.6601, -70.95) knots 5 5 5 5 6 6 6 6
  line L263 (56.6601, -70.95) -> (43.0601, -70.95)
  spline S195 degree 3 poles (43.0601, -70.95) (42.9497, -70.95) (42.8601, -70.8604) (42.8601, -70.75) knots 7 7 7 7 8 8 8 8
  spline S196 degree 3 poles (204.5, -89.8) (204.5, -89.9104) (204.4104, -90) (204.3, -90) knots 0 0 0 0 1 1 1 1
  line L264 (204.3, -90) -> (190.7, -90)
  spline S197 degree 3 poles (190.7, -90) (190.5896, -90) (190.5, -89.9104) (190.5, -89.8) knots 2 2 2 2 3 3 3 3
  line L265 (190.5, -89.8) -> (190.5, -76.2)
  spline S198 degree 3 poles (190.5, -76.2) (190.5, -76.0895) (190.5896, -76) (190.7, -76) knots 4 4 4 4 5 5 5 5
  line L266 (190.7, -76) -> (204.3, -76)
  spline S199 degree 3 poles (204.3, -76) (204.4104, -76) (204.5, -76.0895) (204.5, -76.2) knots 6 6 6 6 7 7 7 7
  line L267 (204.5, -76.2) -> (204.5, -89.8)
  spline S200 degree 3 poles (19.05, 0) (19.05, 0.1105) (19.1396, 0.2) (19.25, 0.2) knots 0 0 0 0 1 1 1 1
  line L268 (19.25, 0.2) -> (32.85, 0.2)
  spline S201 degree 3 poles (32.85, 0.2) (32.9604, 0.2) (33.05, 0.1105) (33.05, 0) knots 2 2 2 2 3 3 3 3
  line L269 (33.05, 0) -> (33.05, -13.6)
  spline S202 degree 3 poles (33.05, -13.6) (33.05, -13.7104) (32.9604, -13.8) (32.85, -13.8) knots 4 4 4 4 5 5 5 5
  line L270 (32.85, -13.8) -> (19.25, -13.8)
  spline S203 degree 3 poles (19.25, -13.8) (19.1396, -13.8) (19.05, -13.7104) (19.05, -13.6) knots 6 6 6 6 7 7 7 7
  line L271 (19.05, -13.6) -> (19.05, 0)
  spline S204 degree 3 poles (38.1, 0) (38.1, 0.1105) (38.1896, 0.2) (38.3, 0.2) knots 0 0 0 0 1 1 1 1
  line L272 (38.3, 0.2) -> (51.9, 0.2)
  spline S205 degree 3 poles (51.9, 0.2) (52.0104, 0.2) (52.1, 0.1105) (52.1, 0) knots 2 2 2 2 3 3 3 3
  line L273 (52.1, 0) -> (52.1, -13.6)
  spline S206 degree 3 poles (52.1, -13.6) (52.1, -13.7104) (52.0104, -13.8) (51.9, -13.8) knots 4 4 4 4 5 5 5 5
  line L274 (51.9, -13.8) -> (38.3, -13.8)
  spline S207 degree 3 poles (38.3, -13.8) (38.1896, -13.8) (38.1, -13.7104) (38.1, -13.6) knots 6 6 6 6 7 7 7 7
  line L275 (38.1, -13.6) -> (38.1, 0)
  line L276 (182.6007, -83.53) -> (181.7758, -83.53)
  line L277 (181.7758, -83.53) -> (181.7758, -89.73)
  line L278 (181.7758, -89.73) -> (179.9508, -89.73)
  line L279 (179.9508, -89.73) -> (179.9508, -90)
  line L280 (179.9508, -90) -> (176.9508, -90)
  line L281 (176.9508, -90) -> (176.9508, -89.73)
  line L282 (176.9508, -89.73) -> (175.1256, -89.73)
  line L283 (175.1256, -89.73) -> (175.1256, -85.25)
  line L284 (175.1256, -85.25) -> (135.4501, -85.25)
  line L285 (135.4501, -85.25) -> (135.4501, -89.8)
  spline S208 degree 3 poles (135.4501, -89.8) (135.4501, -89.9104) (135.3606, -90) (135.2501, -90) knots 10 10 10 10 11 11 11 11
  line L286 (135.2501, -90) -> (121.6501, -90)
  spline S209 degree 3 poles (121.6501, -90) (121.5397, -90) (121.4501, -89.9104) (121.4501, -89.8) knots 12 12 12 12 13 13 13 13
  line L287 (121.4501, -89.8) -> (121.4501, -85.25)
  line L288 (121.4501, -85.25) -> (81.7745, -85.25)
  line L289 (81.7745, -85.25) -> (81.7745, -89.73)
  line L290 (81.7745, -89.73) -> (79.9495, -89.73)
  line L291 (79.9495, -89.73) -> (79.9495, -90)
  line L292 (79.9495, -90) -> (76.9495, -90)
  line L293 (76.9495, -90) -> (76.9495, -89.73)
  line L294 (76.9495, -89.73) -> (75.1244, -89.73)
  line L295 (75.1244, -89.73) -> (75.1244, -83.53)
  line L296 (75.1244, -83.53) -> (74.2993, -83.53)
  line L297 (74.2993, -83.53) -> (74.2993, -80.52)
  line L298 (74.2993, -80.52) -> (75.1244, -80.52)
  line L299 (75.1244, -80.52) -> (75.1244, -77.52)
  line L300 (75.1244, -77.52) -> (81.7743, -77.52)
  spline S210 degree 3 poles (81.7743, -77.52) (81.7743, -77.52) (81.7749, -80.75) (81.7747, -80.75) knots 27 27 27 27 28 28 28 28
  line L301 (81.7747, -80.75) -> (121.4501, -80.75)
  line L302 (121.4501, -80.75) -> (121.4501, -76.2)
  spline S211 degree 3 poles (121.4501, -76.2) (121.4501, -76.0895) (121.5397, -76) (121.6501, -76) knots 30 30 30 30 31 31 31 31
  line L303 (121.6501, -76) -> (135.2501, -76)
  spline S212 degree 3 poles (135.2501, -76) (135.3606, -76) (135.4501, -76.0895) (135.4501, -76.2) knots 32 32 32 32 33 33 33 33
  line L304 (135.4501, -76.2) -> (135.4501, -80.75)
  line L305 (135.4501, -80.75) -> (175.1254, -80.75)
  line L306 (175.1254, -80.75) -> (175.1254, -77.52)
  line L307 (175.1254, -77.52) -> (181.7758, -77.52)
  line L308 (181.7758, -77.52) -> (181.7758, -80.52)
  line L309 (181.7758, -80.52) -> (182.6007, -80.52)
  line L310 (182.6007, -80.52) -> (182.6007, -83.53)
  spline S213 degree 3 poles (25.935, -70.75) (25.935, -70.8604) (25.8456, -70.95) (25.735, -70.95) knots 0 0 0 0 1 1 1 1
  line L311 (25.735, -70.95) -> (12.11, -70.95)
  spline S214 degree 3 poles (12.11, -70.95) (11.9996, -70.95) (11.91, -70.8604) (11.91, -70.75) knots 2 2 2 2 3 3 3 3
  line L312 (11.91, -70.75) -> (11.91, -68.18)
  line L313 (11.91, -68.18) -> (10.2345, -68.18)
  line L314 (10.2345, -68.18) -> (10.2345, -70.68)
  line L315 (10.2345, -70.68) -> (8.4097, -70.68)
  line L316 (8.4097, -70.68) -> (8.4097, -71.93)
  line L317 (8.4097, -71.93) -> (5.4097, -71.93)
  line L318 (5.4097, -71.93) -> (5.4097, -70.68)
  line L319 (5.4097, -70.68) -> (3.5848, -70.68)
  line L320 (3.5848, -70.68) -> (3.5848, -64.48)
  line L321 (3.5848, -64.48) -> (2.7597, -64.48)
  line L322 (2.7597, -64.48) -> (2.7597, -61.47)
  line L323 (2.7597, -61.47) -> (3.5848, -61.47)
  line L324 (3.5848, -61.47) -> (3.5848, -58.47)
  line L325 (3.5848, -58.47) -> (10.2347, -58.47)
  line L326 (10.2347, -58.47) -> (10.2347, -60.97)
  line L327 (10.2347, -60.97) -> (11.91, -60.97)
  line L328 (11.91, -60.97) -> (11.91, -57.15)
  spline S215 degree 3 poles (11.91, -57.15) (11.91, -57.0395) (11.9996, -56.95) (12.11, -56.95) knots 20 20 20 20 21 21 21 21
  line L329 (12.11, -56.95) -> (25.7101, -56.95)
  spline S216 degree 3 poles (25.7101, -56.95) (25.8205, -56.95) (25.91, -57.0395) (25.91, -57.15) knots 22 22 22 22 23 23 23 23
  line L330 (25.91, -57.15) -> (25.91, -60.97)
  line L331 (25.91, -60.97) -> (27.5857, -60.97)
  line L332 (27.5857, -60.97) -> (27.5857, -58.47)
  line L333 (27.5857, -58.47) -> (34.2358, -58.47)
  line L334 (34.2358, -58.47) -> (34.2358, -61.47)
  line L335 (34.2358, -61.47) -> (35.0607, -61.47)
  line L336 (35.0607, -61.47) -> (35.0607, -64.48)
  line L337 (35.0607, -64.48) -> (34.2358, -64.48)
  line L338 (34.2358, -64.48) -> (34.2358, -70.68)
  line L339 (34.2358, -70.68) -> (32.4108, -70.68)
  line L340 (32.4108, -70.68) -> (32.4108, -71.93)
  line L341 (32.4108, -71.93) -> (29.4108, -71.93)
  line L342 (29.4108, -71.93) -> (29.4108, -70.68)
  line L343 (29.4108, -70.68) -> (27.5857, -70.68)
  line L344 (27.5857, -70.68) -> (27.5857, -68.18)
  line L345 (27.5857, -68.18) -> (25.935, -68.18)
  line L346 (25.935, -68.18) -> (25.935, -70.75)
  spline S217 degree 3 poles (76.2, 0) (76.2, 0.1105) (76.2896, 0.2) (76.4, 0.2) knots 0 0 0 0 1 1 1 1
  line L347 (76.4, 0.2) -> (90, 0.2)
  spline S218 degree 3 poles (90, 0.2) (90.1104, 0.2) (90.2, 0.1105) (90.2, 0) knots 2 2 2 2 3 3 3 3
  line L348 (90.2, 0) -> (90.2, -13.6)
  spline S219 degree 3 poles (90.2, -13.6) (90.2, -13.7104) (90.1104, -13.8) (90, -13.8) knots 4 4 4 4 5 5 5 5
  line L349 (90, -13.8) -> (76.4, -13.8)
  spline S220 degree 3 poles (76.4, -13.8) (76.2896, -13.8) (76.2, -13.7104) (76.2, -13.6) knots 6 6 6 6 7 7 7 7
  line L350 (76.2, -13.6) -> (76.2, 0)
  line L351 (0, -13.6) -> (0, 0)
  spline S221 degree 3 poles (0, 0) (0, 0.1105) (0.0896, 0.2) (0.2, 0.2) knots 1 1 1 1 2 2 2 2
  line L352 (0.2, 0.2) -> (13.8, 0.2)
  spline S222 degree 3 poles (13.8, 0.2) (13.9104, 0.2) (14, 0.1105) (14, 0) knots 3 3 3 3 4 4 4 4
  line L353 (14, 0) -> (14, -13.6)
  spline S223 degree 3 poles (14, -13.6) (14, -13.7104) (13.9104, -13.8) (13.8, -13.8) knots 5 5 5 5 6 6 6 6
  line L354 (13.8, -13.8) -> (0.2, -13.8)
  spline S224 degree 3 poles (0.2, -13.8) (0.0896, -13.8) (0, -13.7104) (0, -13.6) knots 7 7 7 7 8 8 8 8
  line L355 (21.1401, -38.1) -> (21.1401, -51.7)
  spline S225 degree 3 poles (21.1401, -51.7) (21.1401, -51.8104) (21.0506, -51.9) (20.9402, -51.9) knots 1 1 1 1 2 2 2 2
  line L356 (20.9402, -51.9) -> (7.3401, -51.9)
  spline S226 degree 3 poles (7.3401, -51.9) (7.2297, -51.9) (7.1401, -51.8104) (7.1401, -51.7) knots 3 3 3 3 4 4 4 4
  line L357 (7.1401, -51.7) -> (7.1401, -38.1)
  spline S227 degree 3 poles (7.1401, -38.1) (7.1401, -37.9895) (7.2297, -37.9) (7.3401, -37.9) knots 5 5 5 5 6 6 6 6
  line L358 (7.3401, -37.9) -> (20.9402, -37.9)
  spline S228 degree 3 poles (20.9402, -37.9) (21.0506, -37.9) (21.1401, -37.9895) (21.1401, -38.1) knots 7 7 7 7 8 8 8 8
  spline S229 degree 3 poles (33.3301, -38.1) (33.3301, -37.9895) (33.4197, -37.9) (33.5301, -37.9) knots 0 0 0 0 1 1 1 1
  line L359 (33.5301, -37.9) -> (47.1301, -37.9)
  spline S230 degree 3 poles (47.1301, -37.9) (47.2405, -37.9) (47.3301, -37.9895) (47.3301, -38.1) knots 2 2 2 2 3 3 3 3
  line L360 (47.3301, -38.1) -> (47.3301, -51.7)
  spline S231 degree 3 poles (47.3301, -51.7) (47.3301, -51.8104) (47.2405, -51.9) (47.1301, -51.9) knots 4 4 4 4 5 5 5 5
  line L361 (47.1301, -51.9) -> (33.5301, -51.9)
  spline S232 degree 3 poles (33.5301, -51.9) (33.4197, -51.9) (33.3301, -51.8104) (33.3301, -51.7) knots 6 6 6 6 7 7 7 7
  line L362 (33.3301, -51.7) -> (33.3301, -38.1)
  spline S233 degree 3 poles (40.15, -89.8) (40.15, -89.9104) (40.0604, -90) (39.95, -90) knots 0 0 0 0 1 1 1 1
  line L363 (39.95, -90) -> (26.35, -90)
  spline S234 degree 3 poles (26.35, -90) (26.2396, -90) (26.15, -89.9104) (26.15, -89.8) knots 2 2 2 2 3 3 3 3
  line L364 (26.15, -89.8) -> (26.15, -76.2)
  spline S235 degree 3 poles (26.15, -76.2) (26.15, -76.0895) (26.2396, -76) (26.35, -76) knots 4 4 4 4 5 5 5 5
  line L365 (26.35, -76) -> (39.95, -76)
  spline S236 degree 3 poles (39.95, -76) (40.0604, -76) (40.15, -76.0895) (40.15, -76.2) knots 6 6 6 6 7 7 7 7
  line L366 (40.15, -76.2) -> (40.15, -89.8)
  spline S237 degree 3 poles (63.9501, -89.8) (63.9501, -89.9104) (63.8605, -90) (63.7501, -90) knots 0 0 0 0 1 1 1 1
  line L367 (63.7501, -90) -> (50.1501, -90)
  spline S238 degree 3 poles (50.1501, -90) (50.0397, -90) (49.9501, -89.9104) (49.9501, -89.8) knots 2 2 2 2 3 3 3 3
  line L368 (49.9501, -89.8) -> (49.9501, -76.2)
  spline S239 degree 3 poles (49.9501, -76.2) (49.9501, -76.0895) (50.0397, -76) (50.1501, -76) knots 4 4 4 4 5 5 5 5
  line L369 (50.1501, -76) -> (63.7501, -76)
  spline S240 degree 3 poles (63.7501, -76) (63.8605, -76) (63.9501, -76.0895) (63.9501, -76.2) knots 6 6 6 6 7 7 7 7
  line L370 (63.9501, -76.2) -> (63.9501, -89.8)
  line L371 (18.7501, -19.05) -> (18.7501, -32.65)
  spline S241 degree 3 poles (18.7501, -32.65) (18.7501, -32.7604) (18.6605, -32.85) (18.5501, -32.85) knots 1 1 1 1 2 2 2 2
  line L372 (18.5501, -32.85) -> (4.9501, -32.85)
  spline S242 degree 3 poles (4.9501, -32.85) (4.8397, -32.85) (4.7501, -32.7604) (4.7501, -32.65) knots 3 3 3 3 4 4 4 4
  line L373 (4.7501, -32.65) -> (4.7501, -19.05)
  spline S243 degree 3 poles (4.7501, -19.05) (4.7501, -18.9395) (4.8397, -18.85) (4.9501, -18.85) knots 5 5 5 5 6 6 6 6
  line L374 (4.9501, -18.85) -> (18.5501, -18.85)
  spline S244 degree 3 poles (18.5501, -18.85) (18.6605, -18.85) (18.7501, -18.9395) (18.7501, -19.05) knots 7 7 7 7 8 8 8 8
  spline S245 degree 3 poles (209.2601, -70.75) (209.2601, -70.8604) (209.1705, -70.95) (209.0601, -70.95) knots 0 0 0 0 1 1 1 1
  line L375 (209.0601, -70.95) -> (195.4601, -70.95)
  spline S246 degree 3 poles (195.4601, -70.95) (195.3497, -70.95) (195.2601, -70.8604) (195.2601, -70.75) knots 2 2 2 2 3 3 3 3
  line L376 (195.2601, -70.75) -> (195.2601, -57.15)
  spline S247 degree 3 poles (195.2601, -57.15) (195.2601, -57.0395) (195.3497, -56.95) (195.4601, -56.95) knots 4 4 4 4 5 5 5 5
  line L377 (195.4601, -56.95) -> (209.0601, -56.95)
  spline S248 degree 3 poles (209.0601, -56.95) (209.1705, -56.95) (209.2601, -57.0395) (209.2601, -57.15) knots 6 6 6 6 7 7 7 7
  line L378 (209.2601, -57.15) -> (209.2601, -70.75)
  spline S249 degree 3 poles (190.2101, -70.75) (190.2101, -70.8604) (190.1205, -70.95) (190.0101, -70.95) knots 0 0 0 0 1 1 1 1
  line L379 (190.0101, -70.95) -> (176.4101, -70.95)
  spline S250 degree 3 poles (176.4101, -70.95) (176.2997, -70.95) (176.2101, -70.8604) (176.2101, -70.75) knots 2 2 2 2 3 3 3 3
  line L380 (176.2101, -70.75) -> (176.2101, -57.15)
  spline S251 degree 3 poles (176.2101, -57.15) (176.2101, -57.0395) (176.2997, -56.95) (176.4101, -56.95) knots 4 4 4 4 5 5 5 5
  line L381 (176.4101, -56.95) -> (190.0101, -56.95)
  spline S252 degree 3 poles (190.0101, -56.95) (190.1205, -56.95) (190.2101, -57.0395) (190.2101, -57.15) knots 6 6 6 6 7 7 7 7
  line L382 (190.2101, -57.15) -> (190.2101, -70.75)
  spline S253 degree 3 poles (16.3501, -89.8) (16.3501, -89.9104) (16.2605, -90) (16.1501, -90) knots 0 0 0 0 1 1 1 1
  line L383 (16.1501, -90) -> (2.5501, -90)
  spline S254 degree 3 poles (2.5501, -90) (2.4396, -90) (2.3501, -89.9104) (2.3501, -89.8) knots 2 2 2 2 3 3 3 3
  line L384 (2.3501, -89.8) -> (2.3501, -76.2)
  spline S255 degree 3 poles (2.3501, -76.2) (2.3501, -76.0895) (2.4396, -76) (2.5501, -76) knots 4 4 4 4 5 5 5 5
  line L385 (2.5501, -76) -> (16.1501, -76)